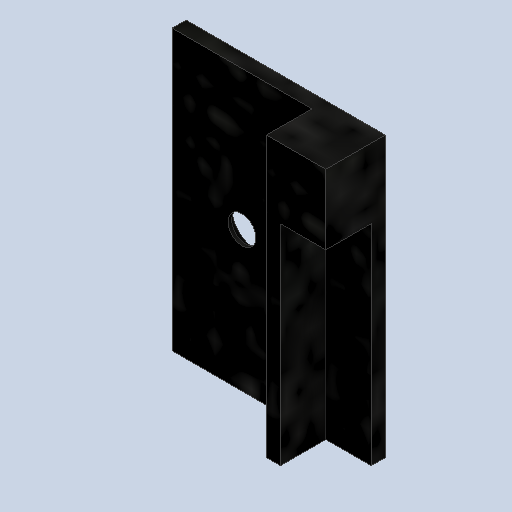
# Autodesk Inventor part: 3DPrintBracket2
Saved by Autodesk Inventor 2022 (Build 260153000, 153)
## iProperties
Created: 2022-11-16
Part Number: 3DPrintBracket2
Material: PC/ABS Plastic
Document SubType Name: Modeling
Designer: braxt
Density: 1.1 g/cm^3
Appearance: Smooth - Black
Description: Formlabs ESD Resin
Stock Number: RS-F2-ESDS-01
Author: braxt
Autodesk Inventor part; units mm, degrees
ref_plane "YZ Plane" through (0, 0, 0) normal (1, 0, 0) x (0, 1, 0)
ref_plane "XZ Plane" through (0, 0, 0) normal (0, 1, 0) x (-1, 0, 0)
ref_plane "XY Plane" through (0, 0, 0) normal (0, 0, 1) x (1, 0, 0)
sketch "Sketch1" plane through (0, 0, 0) normal (0, 1, 0) x (-1, 0, 0)
  line L0 (0, 0) -> (0, 6.5)
  line L1 (0, 0) -> (20, 0)
  line L2 (0, -2) -> (20, -2)
  line L3 (-2, 0) -> (-2, 6.5)
  line L4 (20, -2) -> (20, 0)
  line L5 (-2, 0) -> (-8.5, 0)
  line L6 (-8.5, -2) -> (0, -2)
  line L7 (0, 6.5) -> (-2, 6.5)
  line L8 (-8.5, -2) -> (-8.5, 0)
  dimension "d2" = 20
  dimension "d3" = 2
  dimension "d5" = 2
  dimension "d32" = 6.5
  dimension "d33" = 6.5
  constraints: 18 end point, 3 perpendicular, 2 horizontal, 2 parallel, 1 collinear, 1 vertical
  measures "d2" distance of L0.start L1.end
  measures "d3" distance between parallel lines of L1 L2
  measures "d5" distance between parallel lines of L0 L3
  measures "d32" distance of L3.start L5.end
  measures "d33" distance of L3.start L3.end
extrude "Extrusion1" add sketch "Sketch1" along normal blind 40
sketch "Sketch3" plane through (22, 0, -2) normal (0, 0, -1) x (-1, 0, 0)
  line L0 (42, 0) -> (42, 40) projected
  circle A0 centre (32, 20) radius 3.5
  circle A1 centre (32, 20) radius 2
  line L1 (32, 20) -> (42, 20)
  point P0 (22, 0)
  dimension "d15" = 7
  dimension "d18" = 4
  dimension "d36" = 10
  constraints: 2 centre point, 2 end point, 1 coincident, 1 midpoint
  measures "d15" diameter of A0
  measures "d18" diameter of A1
  measures "d36" distance of L1.start L1.end
hole "Hole1" at (-10, 20, -2) direction (0, 0, 1) diameter 4 end through all countersink diameter 7 countersink angle 90
sketch "Sketch4" plane through (0, 40, 0) normal (0, 1, 0) x (1, 0, 0)
  line L0 (8.5, 2) -> (-20, 2) projected
  line L1 (2, 0) -> (8.5, 0) projected
  line L2 (2, 0) -> (8.5, 0)
  line L3 (8.5, 0) -> (8.5, -6.5)
  line L4 (8.5, -6.5) -> (2, -6.5)
  line L5 (2, -6.5) -> (2, 0)
  point P0 (8.5, 0)
  dimension "d34" = 6.5
  dimension "d35" = 6.5
  constraints: 8 end point, 2 parallel, 1 horizontal, 1 perpendicular
  measures "d34" distance of L3.end L4.end
  measures "d35" distance of L2.end L3.end
extrude "Extrusion4" add sketch "Sketch4" against normal blind 10
body "Solid1"
